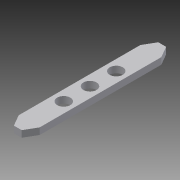
# Autodesk Inventor part: hp_thick_002
Saved by Autodesk Inventor 2014 (Build 180170000, 170)
## iProperties
Created: 2014-03-22
Part Number: hp_thick_002
Material: Generic
Document SubType Name: Modeling
Designer: stephenholtz
Density: 1 g/cm^3
Appearance: Default
Mass: 0.230088 g
Surface Area: 4.57014 cm^2
Volume: 0.230088 cm^3
Author: stephenholtz
Autodesk Inventor part; units mm, degrees
ref_plane "YZ Plane" through (0, 0, 0) normal (1, 0, 0) x (0, 1, 0)
ref_plane "XZ Plane" through (0, 0, 0) normal (0, 1, 0) x (-1, 0, 0)
ref_plane "XY Plane" through (0, 0, 0) normal (0, 0, 1) x (1, 0, 0)
sketch "Sketch1" plane through (0, 0, 0) normal (0, 0, 1) x (1, 0, 0)
  line L0 (-17.4625, -2.54) -> (17.4625, -2.54)
  line L1 (17.4625, -2.54) -> (17.4625, 2.54)
  line L2 (17.4625, 2.54) -> (-17.4625, 2.54)
  line L3 (-17.4625, 2.54) -> (-17.4625, -2.54)
  line L4 (-17.4625, -2.54) -> (17.4625, 2.54) construction
  line L5 (17.4625, -2.54) -> (-17.4625, 2.54) construction
  point P0 (0, 0)
  dimension "bar_length" = 34.925
  dimension "bar_width" = 5.08
  constraints: 12 end point, 2 midpoint, 2 parallel, 1 horizontal, 1 perpendicular
  measures "bar_length" distance of L1.end L2.end
  measures "bar_width" distance of L2.end L0.start
extrude "Extrusion1" add sketch "Sketch1" along normal blind 1.5875
sketch "Sketch2" plane through (0, 0, 1.5875) normal (0, 0, 1) x (1, 0, 0)
  point P0 (0, 0)
  point P1 (0, 0)
  constraints: 1 coincident
hole "Hole1" at (0, 0, 1.5875) direction (0, 0, -1) diameter 3.175 end through all
pattern_linear "Rectangular Pattern1" count 3 spacing 6.35 along (-1, 0, 0) of "Hole1" first direction both ways yes
chamfer "Chamfer2" distance 1.5875 angle 60 1 edges at (17.4625, 2.54, 0.7937) measured on face at (17.4625, 2.04, 0.7938)
chamfer "Chamfer3" distance 1.5875 angle 60 1 edges at (17.4625, -2.54, 0.7937) measured on face at (17.4625, -2.04, 0.7938)
chamfer "Chamfer4" distance 1.5875 angle 60 1 edges at (-17.4625, -2.54, 0.7937) measured on face at (-17.4625, -2.04, 0.7938)
chamfer "Chamfer5" distance 1.5875 angle 60 1 edges at (-17.4625, 2.54, 0.7937) measured on face at (-17.4625, 2.04, 0.7938)
equation "\"d2\" = bar_depth_thick"
equation "\"d6\" = hole_diameter"
equation "\"d15\" = 2 * hole_diameter"
equation "\"bar_depth_thick\" = 1.5875"
equation "\"bar_depth_thin\" = 1.27"
equation "\"hole_diameter\" = 3.175"
body "Solid1"
